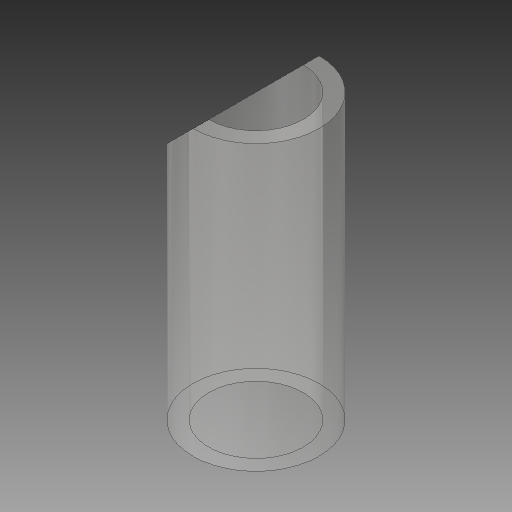
# Autodesk Inventor part: PlexiTubeAnimal
Saved by Autodesk Inventor 2019 (Build 230136000, 136)
## iProperties
Created: 2015-12-01
Part Number: PlexiTubeAnimal
Material: PMMA Plastic
Document SubType Name: Modeling
Designer: Vervaeke-Lab
Mass: 62.7711 g
Surface Area: 244.023 cm^2
Volume: 52.8377 cm^3
Density: 1.188 g/cm^3
Appearance: Polycarbonate - Clear
Author: Vervaeke-Lab
Autodesk Inventor part; units mm, degrees
ref_plane "YZ Plane" through (0, 0, 0) normal (1, 0, 0) x (0, 1, 0)
ref_plane "XZ Plane" through (0, 0, 0) normal (0, 1, 0) x (-1, 0, 0)
ref_plane "XY Plane" through (0, 0, 0) normal (0, 0, 1) x (1, 0, 0)
sketch "Sketch1" plane through (0, 0, 0) normal (0, 1, 0) x (-1, 0, 0)
  circle A0 centre (0, 0) radius 15
  circle A1 centre (0, 0) radius 20
  dimension "d0" = 30
  dimension "d1" = 40
  constraints: 2 centre point, 2 coincident
  measures "d0" diameter of A0
  measures "d1" diameter of A1
extrude "Extrusion1" add sketch "Sketch1" along normal mid plane 90
sketch "Sketch2" plane through (0, 0, 0) normal (0, 0, 1) x (1, 0, 0)
  line L0 (-20, 45) -> (-20, 25)
  line L1 (-20, 25) -> (0, 45)
  line L2 (20, 45) -> (-20, 45) projected
  line L3 (-20, 25) -> (8.2843, 25) construction
  line L4 (0, 45) -> (-20, 45)
  point P0 (0, 0)
  dimension "d7" = 20
  dimension "d9" = 45
  constraints: 8 end point, 1 collinear, 1 equal length, 1 horizontal, 1 midpoint
  measures "d7" distance of L0.start L0.end
  measures "d9" angle of L3 L1
extrude "Extrusion2" cut sketch "Sketch2" along normal through all both and the other way through all
body "Solid1"
